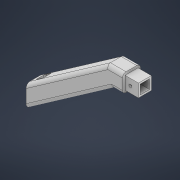
# Autodesk Inventor part: Fahrwerk_rocker_vorne
Saved by Autodesk Inventor 2021 (Build 250183000, 183)
## iProperties
Created: 2020-12-29
Part Number: Fahrwerk_rocker_vorne
Material: Generisch
Document SubType Name: Modeling
Designer: laure
Density: 1 g/cm^3
Appearance: Vorgabe
Author: laure
## iProperties of the stored document _3D-Druck.ipt
Created: 2020-12-30
Part Number: _3D-Druck
Material: Generisch
Document SubType Name: Modeling
Designer: laure
Density: 1 g/cm^3
Appearance: Vorgabe
Author: laure
Autodesk Inventor part; units mm, degrees
ref_plane "YZ Plane" through (0, 0, 0) normal (1, 0, 0) x (0, 1, 0)
ref_plane "XZ Plane" through (0, 0, 0) normal (0, 1, 0) x (-1, 0, 0)
ref_plane "XY Plane" through (0, 0, 0) normal (0, 0, 1) x (1, 0, 0)
sketch "Skizze1" plane through (0, 0, 0) normal (0, 0, 1) x (1, 0, 0)
  line L0 (4.7064, 3.5044) -> (-12.7276, 3.5044)
  line L1 (-12.7276, 3.5044) -> (-102.8343, -59.589)
  line L2 (4.7064, 3.5044) -> (4.7064, -16.4956)
  line L3 (4.7064, -16.4956) -> (-6.4216, -16.4956)
  line L4 (-6.4216, -16.4956) -> (-91.3627, -75.9721)
  line L5 (-102.8343, -59.589) -> (-102.8343, -84.0045)
  line L6 (-102.8343, -84.0045) -> (-91.3627, -75.9721)
  point P0 (0, 0)
  dimension "d0" = 17.434
  dimension "d1" = 110
  dimension "d2" = 145
  dimension "d3" = 20
  dimension "d4" = 20
  dimension "d5" = 11.128
  constraints: 14 end point, 2 vertical, 1 horizontal
  measures "d0" distance of L0.start L0.end
  measures "d1" distance of L0.end L1.end
  measures "d2" angle of L1 L0
  measures "d3" distance of L1.end L4.end
  measures "d4" distance of L0.start L2.end
  measures "d5" distance of L2.end L3.end
extrude "Extrusion1" add sketch "Skizze1" against normal mid plane 20
shell "Wandung1" thickness 2.8 removed faces 2 at (4.7064, -3.1623, -3.3333) at (-102.8343, -67.7275, 3.3333)
ref_plane "Arbeitsebene2" through (4.7064, -12.4956, -10) normal (1, 0, 0) x (0, 0, -1)
sketch "Skizze3" plane through (4.7064, -12.4956, -10) normal (1, 0, 0) x (0, 0, -1)
  line L0 (-3, -65.9356) -> (-3, 0) projected
  line L1 (-17.2, 13.2) -> (-2.8, 13.2)
  line L2 (-2.8, 13.2) -> (-2.8, -1.2)
  line L3 (-2.8, -1.2) -> (-17.2, -1.2)
  line L4 (-17.2, -1.2) -> (-17.2, 13.2)
  line L5 (-4.8, 11.2) -> (-15.2, 11.2)
  line L6 (-15.2, 11.2) -> (-15.2, 0.8)
  line L7 (-15.2, 0.8) -> (-4.8, 0.8)
  line L8 (-4.8, 0.8) -> (-4.8, 11.2)
  line L9 (-2.8, -1.2) -> (-17.2, -1.2) projected
  line L10 (-17.2, -1.2) -> (-17.2, 13.2) projected
  point P0 (-3, -1.2)
  point P1 (-3, 0)
  dimension "d13" = 14.4
  dimension "d14" = 14.4
  dimension "d15" = 2
  dimension "d31" = 0
  dimension "d32" = 0
  constraints: 16 end point, 4 parallel, 2 perpendicular, 1 horizontal, 3 other
  measures "d13" distance of L2.end L3.end
  measures "d14" distance of L1.end L2.end
  measures "d15" distance between parallel lines of L1 L5
  measures "d31" distance between parallel lines of L9 L3
  measures "d32" distance between parallel lines of L10 L4
extrude "Extrusion2" add sketch "Skizze3" along normal blind 15 and the other way blind 7.5
ref_plane "Arbeitsebene1" through (-111.0258, -65.3248, 6) normal (-0.5735764, 0.819152, 0) x (0.819152, 0.5735764, 0)
sketch "Skizze4" plane through (-111.0258, -65.3248, 6) normal (-0.5735764, 0.819152, 0) x (0.819152, 0.5735764, 0)
  line L0 (27, 11) -> (17, 11)
  line L1 (17, 11) -> (17, 1)
  line L2 (17, 1) -> (27, 1)
  line L3 (27, 1) -> (27, 11)
  line L4 (0, 12) -> (0, 0) projected
  line L5 (0, 12) -> (120, 12) projected
  point P0 (128.4158, 6)
  dimension "d21" = 10
  dimension "d22" = 10
  dimension "d23" = 17
  dimension "d24" = 1
  constraints: 8 end point, 2 parallel, 1 horizontal, 1 perpendicular
  measures "d21" distance of L2.end L1.end
  measures "d22" distance of L1.end L0.end
  measures "d23" distance between parallel lines of L1 L4
  measures "d24" distance between parallel lines of L0 L5
extrude "Extrusion3" cut sketch "Skizze4" against normal blind 4
fillet "Rundung3" radius 4 8 edges at (-57.7809, -28.0423, 10) (-57.7809, -28.0423, -10) (-54.6279, -50.2501, 10) (-54.6279, -50.2501, -10) (-0.8576, -16.4956, -10) (-4.0106, 3.5044, -10) (-4.0106, 3.5044, 10) (-0.8576, -16.4956, 10)
fillet "Rundung4" radius 2 4 edges at (-88.1057, -50.9851, -5) (-88.1057, -50.9851, 5) (-96.2972, -56.7208, 5) (-96.2972, -56.7208, -5)
sketch "Skizze5" plane through (-2.7936, -13.6956, 7.2) normal (0, 0, 1) x (1, 0, 0)
  circle A0 centre (13.5, 7.2) radius 1.6
  line L0 (22.5, 14.4) -> (22.5, 0) projected
  line L1 (7.5, 1.2) -> (-4.8892, 1.2) projected
  line L2 (7.5, 0) -> (7.5, 14.4) projected
  point P0 (2.7936, 13.6956)
  dimension "d29" = 3.2
  dimension "d33" = 6
  dimension "d36" = 6
  constraints: 1 centre point
  measures "d29" diameter of A0
  measures "d33" distance from line of L1 A0.centre
  measures "d36" distance from line of L2 A0.centre
extrude "Extrusion4" cut sketch "Skizze5" against normal up to surface (14.4 mm away)
